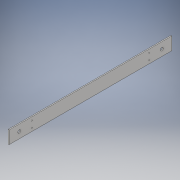
# Autodesk Inventor part: Platte_Kettenglied_unten
Saved by Autodesk Inventor 2018 (Build 220112000, 112)
## iProperties
Created: 2018-01-12
Part Number: Platte_Kettenglied_unten
Material: Generisch
Document SubType Name: Modeling
Designer: Julian
Density: 1 g/cm^3
Appearance: Vorgabe
Author: Julian
Autodesk Inventor part; units mm, degrees
ref_plane "YZ Plane" through (0, 0, 0) normal (1, 0, 0) x (0, 1, 0)
ref_plane "XZ Plane" through (0, 0, 0) normal (0, 1, 0) x (-1, 0, 0)
ref_plane "XY Plane" through (0, 0, 0) normal (0, 0, 1) x (1, 0, 0)
sketch "Skizze1" plane through (0, 0, 0) normal (1, 0, 0) x (0, 1, 0)
  line L0 (0, 0) -> (161.813, 0)
  line L1 (161.813, 0) -> (161.813, 12.7)
  line L2 (161.813, 12.7) -> (0, 12.7)
  line L3 (0, 12.7) -> (0, 0)
  dimension "d0" = 161.813
  dimension "d1" = 12.7
  constraints: 8 end point, 2 parallel, 1 horizontal, 1 perpendicular
  measures "d0" distance of L1.end L2.end
  measures "d1" distance of L0.end L1.end
extrude "Extrusion1" add sketch "Skizze1" along normal blind 1
sketch "Skizze4" plane through (1, 0, 0) normal (1, 0, 0) x (0, 0, -1)
  line L0 (-12.7, 0) -> (0, 0) projected
  line L1 (-6.35, 0) -> (-6.35, 22.5)
  line L2 (-6.35, 0) -> (16.15, 0) construction
  line L3 (-6.35, 22.5) -> (-9.525, 22.5)
  line L4 (-6.35, 22.5) -> (-3.175, 22.5)
  line L5 (0, 161.813) -> (-12.7, 161.813) projected
  line L6 (-6.35, 161.813) -> (-6.35, 139.313)
  line L7 (-6.35, 139.313) -> (-9.525, 139.313)
  line L8 (-6.35, 139.313) -> (-3.175, 139.313)
  dimension "d16" = 22.5
  dimension "d17" = 90
  dimension "d18" = 3.175
  dimension "d19" = 3.175
  dimension "d20" = 22.5
  dimension "d21" = 3.175
  dimension "d22" = 3.175
  constraints: 14 end point, 3 horizontal, 3 perpendicular, 2 midpoint, 2 vertical
  measures "d16" distance of L1.start L1.end
  measures "d17" angle of L2 L1
  measures "d18" distance of L1.end L3.end
  measures "d19" distance of L1.end L4.end
  measures "d20" distance of L6.start L6.end
  measures "d21" distance of L6.end L7.end
  measures "d22" distance of L6.end L8.end
hole "Bohrung2" at (1, 22.5, 9.525) at (1, 22.5, 3.175) at (1, 139.313, 9.525) at (1, 139.313, 3.175) direction (-1, 0, 0) diameter 1 end through all
sketch "Skizze5" plane through (1, 0, 0) normal (1, 0, 0) x (0, 0, -1)
  line L0 (-12.7, 0) -> (0, 0) projected
  line L1 (-6.35, 0) -> (-6.35, 10)
  line L2 (0, 161.813) -> (-12.7, 161.813) projected
  line L3 (-6.35, 161.813) -> (-6.35, 151.813)
  dimension "d30" = 10
  dimension "d31" = 10
  constraints: 4 end point, 2 midpoint, 2 vertical
  measures "d30" distance of L1.start L1.end
  measures "d31" distance of L3.start L3.end
hole "Bohrung3" at (1, 10, 6.35) at (1, 151.813, 6.35) direction (-1, 0, 0) diameter 3 end through all
